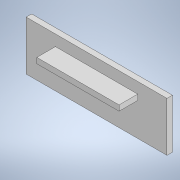
# Autodesk Inventor part: Back Plate
Saved by Autodesk Inventor 2022 (Build 260153000, 153)
## iProperties
Created: 2022-08-19
Part Number: Back Plate
Material: Generic
Document SubType Name: Modeling
Designer: Nick
Density: 1 g/cm^3
Appearance: Default
Author: Nick
Autodesk Inventor part; units mm, degrees
ref_plane "YZ Plane" through (0, 0, 0) normal (1, 0, 0) x (0, 1, 0)
ref_plane "XZ Plane" through (0, 0, 0) normal (0, 1, 0) x (-1, 0, 0)
ref_plane "XY Plane" through (0, 0, 0) normal (0, 0, 1) x (1, 0, 0)
sketch "Sketch1" plane through (0, 0, 0) normal (0, 0, 1) x (1, 0, 0)
  line L0 (0, 0) -> (128.37, 0)
  line L1 (128.37, 0) -> (128.37, 45)
  line L2 (128.37, 45) -> (0, 45)
  line L3 (0, 45) -> (0, 0)
  dimension "d0" = 128.37
  dimension "d1" = 45
  constraints: 8 end point, 2 parallel, 1 horizontal, 1 perpendicular
  measures "d0" distance of L1.end L2.end
  measures "d1" distance of L2.end L0.start
extrude "Extrusion1" add sketch "Sketch1" along normal blind 5
sketch "Sketch2" plane through (0, 0, 5) normal (0, 0, -1) x (-1, 0, 0)
  line L0 (-26.685, 35) -> (-101.685, 35)
  line L1 (-101.685, 35) -> (-101.685, 30)
  line L2 (-101.685, 30) -> (-26.685, 30)
  line L3 (-26.685, 30) -> (-26.685, 35)
  line L4 (-128.37, 45) -> (0, 45) projected
  point P0 (0, 0)
  point P1 (-64.185, 35)
  point P2 (-64.185, 45)
  dimension "d4" = 75
  dimension "d5" = 5
  dimension "d6" = 10
  constraints: 8 end point, 2 midpoint, 2 parallel, 1 horizontal, 1 perpendicular, 1 vertical alignment
  measures "d4" distance of L2.end L1.end
  measures "d5" distance of L1.end L0.end
  measures "d6" distance between parallel lines of L4 L0
extrude "Extrusion2" add sketch "Sketch2" against normal blind 17
body "Solid1"
